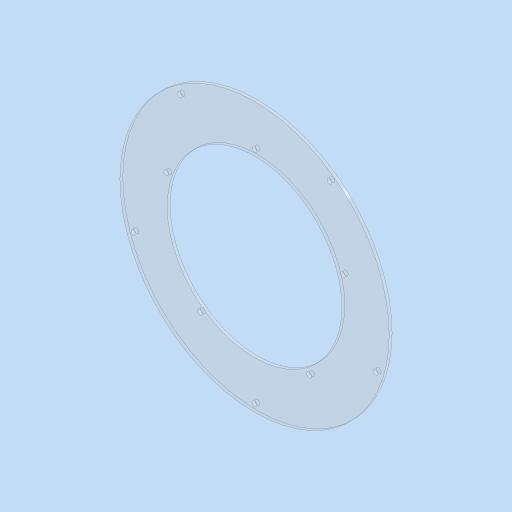
# Autodesk Inventor part: Lid_tight
Saved by Autodesk Inventor 2024.2 (Build 282272000, 272)
## iProperties
Created: 2025-04-30
Part Number: Lid_tight
Material: Generic
Document SubType Name: Modeling
Designer: 23661194
Density: 1 g/cm^3
Appearance: Polycarbonate - Clear
Author: 23661194
Autodesk Inventor part; units mm, degrees
ref_plane "YZ Plane" through (0, 0, 0) normal (1, 0, 0) x (0, 1, 0)
ref_plane "XZ Plane" through (0, 0, 0) normal (0, 1, 0) x (-1, 0, 0)
ref_plane "XY Plane" through (0, 0, 0) normal (0, 0, 1) x (1, 0, 0)
sketch "Sketch1" plane through (0, 0, 0) normal (0, 0, 1) x (1, 0, 0)
  circle A0 centre (0, 0) radius 60
  circle A1 centre (0, 0) radius 92.5
  circle A2 centre (0, 0) radius 63.75
  circle A3 centre (0, 0) radius 87.5
  circle A4 centre (0, 63.75) radius 1.75
  circle A5 centre (-60.6299, 19.6998) radius 1.75
  circle A6 centre (-37.4713, -51.5748) radius 1.75
  circle A7 centre (37.4713, -51.5748) radius 1.75
  circle A8 centre (60.6299, 19.6998) radius 1.75
  line L0 (0, 0) -> (51.4312, 70.789)
  circle A9 centre (51.4312, 70.789) radius 1.75
  line L1 (0, 129.5) -> (0, -129.5) projected
  circle A10 centre (-51.4312, 70.789) radius 1.75
  circle A11 centre (-83.2174, -27.039) radius 1.75
  circle A12 centre (0, -87.5) radius 1.75
  circle A13 centre (83.2174, -27.039) radius 1.75
  dimension "d2" = 127.5
  dimension "d3" = 175
  dimension "d0" = 120
  dimension "d1" = 185
  dimension "d4" = 3.5
  dimension "d7" = 360
  dimension "d9" = 3.5
  dimension "d10" = 36
  dimension "d13" = 360
  constraints: 12 centre point, 5 coincident, 2 end point, 1 point on line, 1 vertical alignment, 27 other
  measures "d0" diameter of A0
  measures "d1" diameter of A1
  measures "d4" diameter of A4
  measures "d9" diameter of A9
  measures "d10" angle of L1 L0
extrude "Extrusion1" add sketch "Sketch1" along normal blind 2 contours A0 L0 A2 A8 A7 L1 | A0 L1 A4 A2 L0 | L1 A2 A6 A5 A4 A0 | L0 A9 A3 A13 A12 L1 A2 A7 A8 | A2 A4 L1 A3 A9 L0 | L1 A12 A3 A11 A10 A4 A2 A5 A6 | A3 L1 A1 A12 A13 A9 | A12 L1 A1 A3 A10 A11
body "Solid1"
